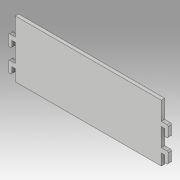
# Autodesk Inventor part: shortside
Saved by Autodesk Inventor 2019.3 (Build 233278000, 278)
## iProperties
Created: 2019-06-26
Part Number: shortside
Material: Generic
Document SubType Name: Modeling
Designer: Dave
Density: 1 g/cm^3
Appearance: Default
Author: Dave
Autodesk Inventor part; units mm, degrees
ref_plane "YZ Plane" through (0, 0, 0) normal (1, 0, 0) x (0, 1, 0)
ref_plane "XZ Plane" through (0, 0, 0) normal (0, 1, 0) x (-1, 0, 0)
ref_plane "XY Plane" through (0, 0, 0) normal (0, 0, 1) x (1, 0, 0)
sketch "Sketch1" plane through (0, 0, 0) normal (0, 0, 1) x (1, 0, 0)
  line L0 (0, 0) -> (64, 0)
  line L1 (64, 50) -> (0, 50)
  line L2 (0, 30) -> (-3, 30)
  line L3 (-3, 30) -> (-3, 25)
  line L4 (-4, 24) -> (-5, 24)
  line L5 (-6, 25) -> (-6, 33)
  line L6 (-5, 34) -> (0, 34)
  line L7 (0, 14) -> (-5, 14)
  line L8 (-6, 13) -> (-6, 5)
  line L9 (-5, 4) -> (-4, 4)
  line L10 (-3, 5) -> (-3, 10)
  line L11 (-3, 10) -> (0, 10)
  arc A0 (-6, 5) -> (-5, 4) centre (-5, 5) ccw
  arc A1 (-4, 4) -> (-3, 5) centre (-4, 5) ccw
  arc A2 (-5, 14) -> (-6, 13) centre (-5, 13) ccw
  arc A3 (-6, 25) -> (-5, 24) centre (-5, 25) ccw
  arc A4 (-4, 24) -> (-3, 25) centre (-4, 25) ccw
  arc A5 (-5, 34) -> (-6, 33) centre (-5, 33) ccw
  line L12 (64, 50) -> (64, 0) construction
  line L13 (128, 0) -> (64, 0)
  line L14 (64, 50) -> (128, 50)
  line L15 (128, 30) -> (131, 30)
  line L16 (131, 30) -> (131, 25)
  line L17 (132, 24) -> (133, 24)
  line L18 (134, 25) -> (134, 33)
  line L19 (133, 34) -> (128, 34)
  line L20 (128, 14) -> (133, 14)
  line L21 (134, 13) -> (134, 5)
  line L22 (133, 4) -> (132, 4)
  line L23 (131, 5) -> (131, 10)
  line L24 (131, 10) -> (128, 10)
  arc A6 (133, 4) -> (134, 5) centre (133, 5) ccw
  arc A7 (131, 5) -> (132, 4) centre (132, 5) ccw
  arc A8 (134, 13) -> (133, 14) centre (133, 13) ccw
  arc A9 (133, 24) -> (134, 25) centre (133, 25) ccw
  arc A10 (131, 25) -> (132, 24) centre (132, 25) ccw
  arc A11 (134, 33) -> (133, 34) centre (133, 33) ccw
  line L25 (0, 50) -> (0, 34)
  line L26 (0, 30) -> (0, 14)
  line L27 (0, 10) -> (0, 0)
  line L28 (128, 50) -> (128, 34)
  line L29 (128, 30) -> (128, 14)
  line L30 (128, 10) -> (128, 0)
  point P0 (-3, 24)
  point P1 (-6, 24)
  point P2 (-6, 34)
  point P3 (-6, 14)
  point P4 (-6, 4)
  point P5 (-3, 4)
  point P6 (-2.5, 14)
  point P7 (131, 24)
  point P8 (134, 24)
  point P9 (134, 34)
  point P10 (134, 14)
  point P11 (134, 4)
  point P12 (131, 4)
  point P13 (130.5, 14)
  dimension "d0" = 10
  dimension "d1" = 4
  dimension "d2" = 3
  dimension "d6" = 10
  dimension "d7" = 4
  dimension "d8" = 30
  dimension "d9" = 50
  dimension "d11" = 1
  dimension "d12" = 64
  dimension "d13" = 64
  dimension "d14" = 6
  dimension "d15" = 6
  constraints: 62 end point, 33 symmetric about line, 32 point on line, 24 point on circle, 13 perpendicular, 13 tangent, 12 centre point, 5 equal radius, 2 horizontal, 1 collinear, 1 midpoint, 1 parallel, 6 other
  measures "d0" distance of point (-6, 24) point (-6, 34)
  measures "d1" distance between parallel lines of L2 L6
  measures "d2" distance of point (-3, 24) point (-6, 24)
  measures "d6" distance between parallel lines of L0 L11
  measures "d7" distance between parallel lines of L11 L7
  measures "d8" distance between parallel lines of L0 L2
  measures "d9" distance of L1.end L0.start
  measures "d11" radius of A0
  measures "d12" distance of L1.start L1.end
  measures "d13" distance of L0.start L0.end
  measures "d14" distance between parallel lines of L18 L28
  measures "d15" distance between parallel lines of L18 L29
extrude "Extrusion1" add sketch "Sketch1" along normal blind 3
body "Solid1"
